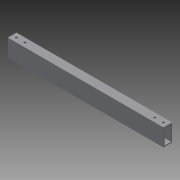
# Autodesk Inventor part: 2x1 boxbeam 18 in
Saved by Autodesk Inventor 2015 (Build 190159000, 159)
## iProperties
Created: 2015-01-21
Part Number: 2x1 boxbeam 18 in
Material: Generic
Document SubType Name: Modeling
Designer: chapale16
Density: 1 g/cm^3
Appearance: Default
Author: chapale16
Autodesk Inventor part; units mm, degrees
ref_plane "YZ Plane" through (0, 0, 0) normal (1, 0, 0) x (0, 1, 0)
ref_plane "XZ Plane" through (0, 0, 0) normal (0, 1, 0) x (-1, 0, 0)
ref_plane "XY Plane" through (0, 0, 0) normal (0, 0, 1) x (1, 0, 0)
sketch "Sketch1" plane through (0, 0, 0) normal (1, 0, 0) x (0, 1, 0)
  line L0 (0, 0) -> (50.8, 0)
  line L1 (50.8, 0) -> (50.8, -25.4)
  line L2 (50.8, -25.4) -> (0, -25.4)
  line L3 (0, -25.4) -> (0, 0)
  line L4 (47.625, -22.225) -> (47.625, -3.175)
  line L5 (47.625, -3.175) -> (3.175, -3.175)
  line L6 (3.175, -3.175) -> (3.175, -22.225)
  line L7 (3.175, -22.225) -> (47.625, -22.225)
  dimension "d0" = 50.8
  dimension "d1" = 25.4
  dimension "d2" = 3.175
  constraints: 16 end point, 4 parallel, 2 perpendicular, 1 horizontal, 3 other
  measures "d0" distance of L1.end L2.end
  measures "d1" distance of L0.end L1.end
  measures "d2" distance between parallel lines of L1 L4
extrude "Extrusion1" add sketch "Sketch1" along normal blind 457.2
sketch "Sketch2" plane through (0, 50.8, 0) normal (0, 1, 0) x (1, 0, 0)
  circle A0 centre (419.1, -332.2693) radius 3.175 projected
  circle A1 centre (444.5, -332.2693) radius 3.175 projected
  circle A2 centre (469.9, -281.4693) radius 3.175 projected
  circle A3 centre (469.9, -306.8693) radius 3.175 projected
  circle A4 centre (469.9, -357.6693) radius 3.175 projected
  circle A5 centre (469.9, -383.0693) radius 3.175 projected
  circle A6 centre (469.9, -332.2693) radius 3.175 projected
  line L0 (481.0125, -276.7068) -> (477.8375, -273.5318) projected
  line L1 (477.8375, -273.5318) -> (461.9625, -273.5318) projected
  line L2 (461.9625, -273.5318) -> (458.7875, -276.7068) projected
  line L3 (458.7875, -276.7068) -> (458.7875, -295.7568) projected
  arc A7 (433.3875, -321.1568) -> (458.7875, -295.7568) centre (433.3875, -295.7568) ccw projected
  line L4 (433.3875, -321.1568) -> (414.3375, -321.1568) projected
  line L5 (414.3375, -321.1568) -> (411.1625, -324.3318) projected
  line L6 (411.1625, -324.3318) -> (411.1625, -340.2068) projected
  line L7 (411.1625, -340.2068) -> (414.3375, -343.3818) projected
  line L8 (414.3375, -343.3818) -> (433.3875, -343.3818) projected
  arc A8 (458.7875, -368.7818) -> (433.3875, -343.3818) centre (433.3875, -368.7818) ccw projected
  line L9 (458.7875, -368.7818) -> (458.7875, -387.8318) projected
  line L10 (458.7875, -387.8318) -> (461.9625, -391.0068) projected
  line L11 (461.9625, -391.0068) -> (477.8375, -391.0068) projected
  line L12 (477.8375, -391.0068) -> (481.0125, -387.8318) projected
  line L13 (481.0125, -387.8318) -> (481.0125, -276.7068) projected
  circle A9 centre (38.1, -332.2693) radius 3.175 projected
  circle A10 centre (12.7, -332.2693) radius 3.175 projected
  circle A11 centre (-12.7, -281.4693) radius 3.175 projected
  circle A12 centre (-12.7, -306.8693) radius 3.175 projected
  circle A13 centre (-12.7, -357.6693) radius 3.175 projected
  circle A14 centre (-12.7, -383.0693) radius 3.175 projected
  circle A15 centre (-12.7, -332.2693) radius 3.175 projected
  line L14 (-23.8125, -276.7068) -> (-20.6375, -273.5318) projected
  line L15 (-23.8125, -387.8318) -> (-23.8125, -276.7068) projected
  line L16 (-20.6375, -391.0068) -> (-23.8125, -387.8318) projected
  line L17 (-4.7625, -391.0068) -> (-20.6375, -391.0068) projected
  line L18 (-1.5875, -387.8318) -> (-4.7625, -391.0068) projected
  line L19 (-1.5875, -368.7818) -> (-1.5875, -387.8318) projected
  arc A16 (23.8125, -343.3818) -> (-1.5875, -368.7818) centre (23.8125, -368.7818) ccw projected
  line L20 (42.8625, -343.3818) -> (23.8125, -343.3818) projected
  line L21 (46.0375, -340.2068) -> (42.8625, -343.3818) projected
  line L22 (46.0375, -324.3318) -> (46.0375, -340.2068) projected
  line L23 (42.8625, -321.1568) -> (46.0375, -324.3318) projected
  line L24 (23.8125, -321.1568) -> (42.8625, -321.1568) projected
  arc A17 (-1.5875, -295.7568) -> (23.8125, -321.1568) centre (23.8125, -295.7568) ccw projected
  line L25 (-1.5875, -276.7068) -> (-1.5875, -295.7568) projected
  line L26 (-4.7625, -273.5318) -> (-1.5875, -276.7068) projected
  line L27 (-20.6375, -273.5318) -> (-4.7625, -273.5318) projected
  circle A18 centre (419.1, 12.7) radius 3.175 projected
  circle A19 centre (444.5, 12.7) radius 3.175 projected
  circle A20 centre (469.9, -38.1) radius 3.175 projected
  circle A21 centre (469.9, -12.7) radius 3.175 projected
  circle A22 centre (469.9, 38.1) radius 3.175 projected
  circle A23 centre (469.9, 63.5) radius 3.175 projected
  circle A24 centre (469.9, 12.7) radius 3.175 projected
  line L28 (481.0125, -42.8625) -> (477.8375, -46.0375) projected
  line L29 (481.0125, 68.2625) -> (481.0125, -42.8625) projected
  line L30 (477.8375, 71.4375) -> (481.0125, 68.2625) projected
  line L31 (461.9625, 71.4375) -> (477.8375, 71.4375) projected
  line L32 (458.7875, 68.2625) -> (461.9625, 71.4375) projected
  line L33 (458.7875, 49.2125) -> (458.7875, 68.2625) projected
  arc A25 (433.3875, 23.8125) -> (458.7875, 49.2125) centre (433.3875, 49.2125) ccw projected
  line L34 (414.3375, 23.8125) -> (433.3875, 23.8125) projected
  line L35 (411.1625, 20.6375) -> (414.3375, 23.8125) projected
  line L36 (411.1625, 4.7625) -> (411.1625, 20.6375) projected
  line L37 (414.3375, 1.5875) -> (411.1625, 4.7625) projected
  line L38 (433.3875, 1.5875) -> (414.3375, 1.5875) projected
  arc A26 (458.7875, -23.8125) -> (433.3875, 1.5875) centre (433.3875, -23.8125) ccw projected
  line L39 (458.7875, -42.8625) -> (458.7875, -23.8125) projected
  line L40 (461.9625, -46.0375) -> (458.7875, -42.8625) projected
  line L41 (477.8375, -46.0375) -> (461.9625, -46.0375) projected
  circle A27 centre (38.1, 12.7) radius 3.175 projected
  circle A28 centre (12.7, 12.7) radius 3.175 projected
  circle A29 centre (-12.7, -38.1) radius 3.175 projected
  circle A30 centre (-12.7, -12.7) radius 3.175 projected
  circle A31 centre (-12.7, 38.1) radius 3.175 projected
  circle A32 centre (-12.7, 63.5) radius 3.175 projected
  circle A33 centre (-12.7, 12.7) radius 3.175 projected
  line L42 (-23.8125, -42.8625) -> (-20.6375, -46.0375) projected
  line L43 (-20.6375, -46.0375) -> (-4.7625, -46.0375) projected
  line L44 (-4.7625, -46.0375) -> (-1.5875, -42.8625) projected
  line L45 (-1.5875, -42.8625) -> (-1.5875, -23.8125) projected
  arc A34 (23.8125, 1.5875) -> (-1.5875, -23.8125) centre (23.8125, -23.8125) ccw projected
  line L46 (23.8125, 1.5875) -> (42.8625, 1.5875) projected
  line L47 (42.8625, 1.5875) -> (46.0375, 4.7625) projected
  line L48 (46.0375, 4.7625) -> (46.0375, 20.6375) projected
  line L49 (46.0375, 20.6375) -> (42.8625, 23.8125) projected
  line L50 (42.8625, 23.8125) -> (23.8125, 23.8125) projected
  arc A35 (-1.5875, 49.2125) -> (23.8125, 23.8125) centre (23.8125, 49.2125) ccw projected
  line L51 (-1.5875, 49.2125) -> (-1.5875, 68.2625) projected
  line L52 (-1.5875, 68.2625) -> (-4.7625, 71.4375) projected
  line L53 (-4.7625, 71.4375) -> (-20.6375, 71.4375) projected
  line L54 (-20.6375, 71.4375) -> (-23.8125, 68.2625) projected
  line L55 (-23.8125, 68.2625) -> (-23.8125, -42.8625) projected
  point P0 (0, 0)
extrude "Extrusion2" cut sketch "Sketch2" against normal blind 50.8 contours A18 | A19 | A27 | A28
body "Solid1"
